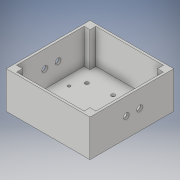
# Autodesk Inventor part: 546-1590YFLBK-ADL5534
Saved by Autodesk Inventor 2018 (Build 220112000, 112)
## iProperties
Created: 2018-04-27
Part Number: 546-1590YFLBK-ADL5534
Material: Generic
Document SubType Name: Modeling
Designer: bbramman
Density: 1 g/cm^3
Appearance: Default
Author: bbramman
Autodesk Inventor part; units mm, degrees
ref_plane "YZ Plane" through (0, 0, 0) normal (1, 0, 0) x (0, 1, 0)
ref_plane "XZ Plane" through (0, 0, 0) normal (0, 1, 0) x (-1, 0, 0)
ref_plane "XY Plane" through (0, 0, 0) normal (0, 0, 1) x (1, 0, 0)
sketch "Sketch1" plane through (0, 0, 0) normal (0, 1, 0) x (-1, 0, 0)
  line L0 (45.9867, -45.9867) -> (-45.9867, -45.9867)
  line L1 (-45.9867, -45.9867) -> (-45.9867, 45.9867)
  line L2 (-45.9867, 45.9867) -> (45.9867, 45.9867)
  line L3 (45.9867, 45.9867) -> (45.9867, -45.9867)
  line L4 (45.9867, -45.9867) -> (-45.9867, 45.9867) construction
  line L5 (-45.9867, -45.9867) -> (45.9867, 45.9867) construction
  point P0 (0, 0)
  dimension "d0" = 91.9734
  dimension "d1" = 91.9734
  constraints: 12 end point, 2 midpoint, 2 parallel, 1 horizontal, 1 perpendicular
  measures "d0" distance of L1.end L2.end
  measures "d1" distance of L0.end L1.end
extrude "Extrusion1" add sketch "Sketch1" along normal blind 2.4892
sketch "Sketch2" plane through (0, 2.4892, 0) normal (0, 1, 0) x (1, 0, 0)
  line L0 (-45.9867, -45.9867) -> (45.9867, -45.9867) projected
  line L1 (45.9867, 45.9867) -> (-45.9867, 45.9867) projected
  line L2 (-45.9867, -45.9867) -> (45.9867, -45.9867)
  line L3 (45.9867, -45.9867) -> (45.9867, 45.9867)
  line L4 (45.9867, 45.9867) -> (-45.9867, 45.9867)
  line L5 (-45.9867, 45.9867) -> (-45.9867, -45.9867)
  line L6 (43.4975, -43.4975) -> (-43.4975, 43.4975) construction
  line L7 (-43.4975, -43.4975) -> (43.4975, 43.4975) construction
  line L8 (-45.9867, -45.9867) -> (-36.9951, -45.9867)
  line L9 (-45.9867, -36.9951) -> (-45.9867, -45.9867)
  line L10 (-45.9867, 45.9867) -> (-45.9867, -45.9867) projected
  line L11 (-45.9867, 45.9867) -> (-36.9951, 45.9867)
  line L12 (-45.9867, 36.9951) -> (-45.9867, 45.9867)
  line L13 (45.9867, 45.9867) -> (36.9951, 45.9867)
  line L14 (45.9867, 36.9951) -> (45.9867, 45.9867)
  line L15 (45.9867, -45.9867) -> (36.9951, -45.9867)
  line L16 (45.9867, -36.9951) -> (45.9867, -45.9867)
  line L17 (-36.9951, -43.4975) -> (-36.9951, -36.9951)
  line L18 (-36.9951, -36.9951) -> (-43.4975, -36.9951)
  line L19 (-43.4975, 36.9951) -> (-36.9951, 36.9951)
  line L20 (-36.9951, 36.9951) -> (-36.9951, 43.4975)
  line L21 (36.9951, 36.9951) -> (43.4975, 36.9951)
  line L22 (36.9951, 43.4975) -> (36.9951, 36.9951)
  line L23 (43.4975, -36.9951) -> (36.9951, -36.9951)
  line L24 (36.9951, -36.9951) -> (36.9951, -43.4975)
  line L25 (-36.9951, -43.4975) -> (36.9951, -43.4975)
  line L26 (43.4975, -36.9951) -> (43.4975, 36.9951)
  line L27 (36.9951, 43.4975) -> (-36.9951, 43.4975)
  line L28 (-43.4975, 36.9951) -> (-43.4975, -36.9951)
  point P0 (0, 0)
  dimension "d4" = 86.995
  dimension "d5" = 86.995
  dimension "d6" = 8.9916
  dimension "d7" = 8.9916
  dimension "d10" = 8.9916
  dimension "d11" = 8.9916
  constraints: 52 end point, 7 horizontal, 5 perpendicular, 2 midpoint, 2 parallel
  measures "d4" distance of L6.end L7.end
  measures "d5" distance of L7.start L6.end
  measures "d6" distance of L9.start L17.end
  measures "d7" distance of L17.end L8.end
  measures "d10" distance of L14.start L21.start
  measures "d11" distance of L21.start L13.end
extrude "Extrusion2" add sketch "Sketch2" along normal blind 37.9984
sketch "Sketch3" plane through (0, 2.4892, 0) normal (0, 1, 0) x (1, 0, 0)
  line L0 (25.9969, -22.5044) -> (-25.9969, 22.5044) construction
  line L1 (-25.9969, -22.5044) -> (25.9969, 22.5044) construction
  circle A0 centre (-25.9969, -22.5044) radius 1.9939
  circle A1 centre (-25.9969, 22.5044) radius 1.9939
  circle A2 centre (25.9969, 22.5044) radius 1.9939
  circle A3 centre (25.9969, -22.5044) radius 1.9939
  line L2 (32.9946, -9.9949) -> (-32.9946, 9.9949) construction
  line L3 (-32.9946, -9.9949) -> (32.9946, 9.9949) construction
  circle A4 centre (-32.9946, -9.9949) radius 1.4986
  circle A5 centre (-32.9946, 9.9949) radius 1.4986
  circle A6 centre (32.9946, -9.9949) radius 1.4986
  circle A7 centre (32.9946, 9.9949) radius 1.4986
  circle A8 centre (0, -25.4) radius 2.0828
  circle A9 centre (0, 25.4) radius 2.0828
  point P0 (0, 0)
  dimension "d16" = 51.9938
  dimension "d17" = 45.0088
  dimension "d18" = 3.9878
  dimension "d19" = 3.9878
  dimension "d20" = 3.9878
  dimension "d21" = 3.9878
  dimension "d22" = 65.9892
  dimension "d23" = 19.9898
  dimension "d24" = 2.9972
  dimension "d25" = 2.9972
  dimension "d26" = 2.9972
  dimension "d27" = 2.9972
  dimension "d30" = 4.1656
  dimension "d31" = 4.1656
  constraints: 10 centre point, 8 coincident, 8 end point, 4 midpoint
  measures "d16" distance of L0.end L1.end
  measures "d17" distance of L1.start L0.end
  measures "d18" diameter of A0
  measures "d19" diameter of A1
  measures "d20" diameter of A2
  measures "d21" diameter of A3
  measures "d22" distance of L2.end L3.end
  measures "d23" distance of L3.start L2.end
  measures "d24" diameter of A4
  measures "d25" diameter of A5
  measures "d26" diameter of A6
  measures "d27" diameter of A7
  measures "d30" diameter of A8
  measures "d31" diameter of A9
extrude "Extrusion3" cut sketch "Sketch3" against normal through all
sketch "Sketch4" plane through (-43.4975, 2.4892, 36.9951) normal (1, 0, 0) x (0, 0, -1)
  line L0 (0, 0) -> (0, 37.9984) projected
  line L1 (0, 19.05) -> (9.4996, 19.05)
  line L2 (0, 19.05) -> (9.4996, 19.05) construction
  line L3 (9.4996, 19.05) -> (30.7594, 19.05)
  line L4 (30.7594, 19.05) -> (45.4406, 19.05)
  circle A0 centre (30.7594, 19.05) radius 3.175
  circle A1 centre (45.4406, 19.05) radius 3.175
  point P0 (36.9951, -2.4892)
  point P1 (73.9902, 0)
  dimension "d44" = 9.4996
  dimension "d45" = 0
  dimension "d46" = 21.2598
  dimension "d47" = 14.6812
  dimension "d48" = 6.35
  dimension "d49" = 6.35
  constraints: 8 end point, 2 centre point, 2 coincident, 2 horizontal, 2 point on line, 1 collinear, 1 perpendicular
  measures "d44" distance of L1.start L1.end
  measures "d45" distance between parallel lines of L1 L2
  measures "d46" distance of L2.end L3.end
  measures "d47" distance of L3.end L4.end
  measures "d48" diameter of A0
  measures "d49" diameter of A1
extrude "Extrusion4" cut sketch "Sketch4" against normal through all
sketch "Sketch5" plane through (43.4975, 2.4892, -36.9951) normal (-1, 0, 0) x (0, 0, 1)
  line L0 (73.9902, 0) -> (73.9902, 37.9984) projected
  line L1 (73.9902, 19.05) -> (64.4906, 19.05)
  line L2 (64.4906, 19.05) -> (43.2308, 19.05)
  line L3 (43.2308, 19.05) -> (28.5496, 19.05)
  circle A0 centre (43.2308, 19.05) radius 3.175
  circle A1 centre (28.5496, 19.05) radius 3.175
  point P0 (36.9951, -2.4892)
  point P1 (0, 37.9984)
  dimension "d50" = 9.4996
  dimension "d51" = 21.2598
  dimension "d52" = 14.6812
  dimension "d53" = 6.35
  dimension "d54" = 6.35
  constraints: 6 end point, 2 centre point, 2 coincident, 2 horizontal, 2 point on line
  measures "d50" distance of L1.start L1.end
  measures "d51" distance of L1.end L2.end
  measures "d52" distance of L2.end L3.end
  measures "d53" diameter of A0
  measures "d54" diameter of A1
extrude "Extrusion5" cut sketch "Sketch5" against normal through all
body "Solid1"
